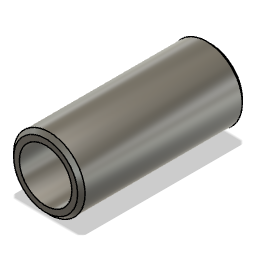
Tilt Bracket Shaft v2 (Autodesk Fusion 360 design; units mm, degrees)
Autodesk Fusion 360 part; units mm, degrees
sketch "Sketch1" plane through (0, 0, 0) normal (0, 0, 1) x (1, 0, 0)
  circle A0 centre (0, 0) radius 2.3813
  circle A1 centre (0, 0) radius 1.75
  dimension "d1" = 4.7625
  dimension "d2" = 3.5
  constraint coincident A0.centre A1.centre
  constraint concentric A0 A1
  measures "d1" diameter of A0
  measures "d2" diameter of A1
extrude "Extrude1" add sketch "Sketch1" along normal mid plane 11
chamfer "Chamfer1" distance 0.25 angle 45 2 edges at (-2.2201, 0.8611, -5.5) (-2.2201, -0.8611, 5.5)
